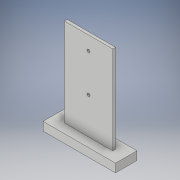
# Autodesk Inventor part: Middle Frame
Saved by Autodesk Inventor 2017 (Build 210142000, 142)
## iProperties
Created: 2018-03-04
Part Number: Middle Frame
Material: Generic
Document SubType Name: Modeling
Designer: Russ
Density: 1 g/cm^3
Appearance: Default
Author: Russ
Autodesk Inventor part; units mm, degrees
ref_plane "YZ Plane" through (0, 0, 0) normal (1, 0, 0) x (0, 1, 0)
ref_plane "XZ Plane" through (0, 0, 0) normal (0, 1, 0) x (-1, 0, 0)
ref_plane "XY Plane" through (0, 0, 0) normal (0, 0, 1) x (1, 0, 0)
sketch "Sketch1" plane through (0, 0, 0) normal (0, 0, 1) x (1, 0, 0)
  circle A0 centre (0, 0) radius 7.62
  circle A1 centre (0, -40.005) radius 30.48
  circle A2 centre (0, 0) radius 1.55
  circle A3 centre (0, -40.005) radius 1.55
  line L0 (-25.4, 14.478) -> (25.4, 14.478)
  line L1 (25.4, 14.478) -> (25.4, -78.232)
  line L2 (25.4, -87.122) -> (-25.4, -87.122)
  line L3 (-25.4, -78.232) -> (-25.4, 14.478)
  line L4 (-25.4, -87.122) -> (-38.1, -87.122)
  line L5 (-38.1, -87.122) -> (-38.1, -78.232)
  line L6 (-38.1, -78.232) -> (-25.4, -78.232)
  line L7 (25.4, -87.122) -> (38.1, -87.122)
  line L8 (38.1, -87.122) -> (38.1, -78.232)
  line L9 (38.1, -78.232) -> (25.4, -78.232)
  dimension "d0" = 40.005
  dimension "d1" = 15.24
  dimension "d2" = 60.96
  dimension "d3" = 3.1
  dimension "d4" = 3.1
  dimension "d5" = 14.478
  dimension "d6" = 25.4
  dimension "d7" = 25.4
  dimension "d8" = 101.6
  dimension "d9" = 12.7
  dimension "d10" = 12.7
  dimension "d11" = 8.89
  constraints: 20 end point, 4 centre point, 4 perpendicular, 3 coincident, 3 point on line, 2 horizontal, 2 parallel
  measures "d0" distance of A1.centre point (0, 0)
  measures "d1" diameter of A0
  measures "d2" diameter of A1
  measures "d3" diameter of A2
  measures "d4" diameter of A3
  measures "d5" distance from line of L0 point (0, 0)
  measures "d6" distance from line of point (0, 0) L1
  measures "d7" distance from line of A2.centre L3
  measures "d8" distance of L1.start L2.start
  measures "d9" distance between parallel lines of L8 L1
  measures "d10" distance between parallel lines of L3 L5
  measures "d11" distance of L4.end L6.start
extrude "Extrusion1" add sketch "Sketch1" along normal blind 3 contours A0 | L1 A1 L3 | A1 L3 L0 L1 | L1 L9 L8 L7 L2 L4 L5 L6 L3 A1
sketch "Sketch2" plane through (38.1, -87.122, 0) normal (1, 0, 0) x (0, 0, -1)
  line L0 (0, 8.89) -> (-3, 8.89) projected
  line L1 (0, 0) -> (-3, 0) projected
  line L2 (-1.5, 8.89) -> (9.8044, 8.89)
  line L3 (9.8044, 8.89) -> (9.8044, 0)
  line L4 (9.8044, 0) -> (-1.5, 0)
  line L5 (-1.5, 0) -> (-1.5, 8.89)
  line L6 (-1.5, 8.89) -> (-12.81, 8.89)
  line L7 (-12.81, 8.89) -> (-12.81, 0)
  line L8 (-12.81, 0) -> (-1.5, 0)
  line L9 (-1.5, 0) -> (-1.5, 8.89)
  line L10 (-3, 0) -> (-3, 8.89) projected
  line L11 (-3, 8.89) -> (-3, 0)
  line L12 (0, 0) -> (0, 8.89) projected
  line L13 (0, 8.89) -> (0, 0)
  point P0 (0, 87.122)
  dimension "d15" = 8.89
  dimension "d19" = 9.81
  dimension "d20" = 9.8044
  constraints: 20 end point, 4 parallel, 4 perpendicular, 2 horizontal, 1 midpoint, 1 point on line
  measures "d15" distance of L2.end L3.end
  measures "d19" distance between parallel lines of L10 L7
  measures "d20" distance between parallel lines of L3 L12
extrude "Extrusion2" add sketch "Sketch2" against normal blind 76.2
body "Solid1"
